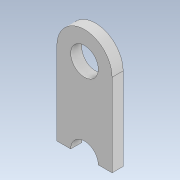
# Autodesk Inventor part: MainDrive_Abstandhilfe
Saved by Autodesk Inventor 2022 (Build 260153000, 153)
## iProperties
Created: 2022-10-10
Part Number: MainDrive_Abstandhilfe
Material: Generisch
Document SubType Name: Modeling
Designer: alexw
Density: 1 g/cm^3
Appearance: Vorgabe
Author: alexw
Autodesk Inventor part; units mm, degrees
ref_plane "YZ Plane" through (0, 0, 0) normal (1, 0, 0) x (0, 1, 0)
ref_plane "XZ Plane" through (0, 0, 0) normal (0, 1, 0) x (-1, 0, 0)
ref_plane "XY Plane" through (0, 0, 0) normal (0, 0, 1) x (1, 0, 0)
sketch "Skizze1" plane through (0, 0, 0) normal (0, 0, 1) x (1, 0, 0)
  circle A0 centre (0, 0) radius 5 construction
  line L0 (-5, 0) -> (-10, 0)
  line L1 (-10, 0) -> (-10, 30)
  arc A1 (10, 30) -> (-10, 30) centre (0, 30) ccw
  line L2 (10, 30) -> (10, 0)
  line L3 (10, 0) -> (5, 0)
  arc A2 (5, 0) -> (-5, -0.0088) centre (0, 0) ccw
  line L4 (0, 0) -> (5, 0) construction
  circle A3 centre (0, 30) radius 5
  dimension "d0" = 10
  dimension "d1" = 30
  dimension "d2" = 20
  dimension "d3" = 10
  constraints: 10 end point, 8 point on circle, 4 centre point, 3 tangent, 2 coincident, 2 collinear, 2 horizontal, 2 point on line, 1 parallel, 1 perpendicular
  measures "d0" diameter of A0
  measures "d1" distance of A1.centre point (0, 0)
  measures "d2" distance between parallel lines of L2 L1
  measures "d3" diameter of A3
extrude "Extrusion1" add sketch "Skizze1" along normal blind 4
